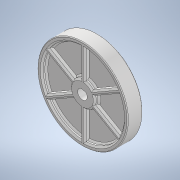
# Autodesk Inventor part: Test Gear
Saved by Autodesk Inventor 2020.2 (Build 242310000, 310)
## iProperties
Created: 2020-04-13
Part Number: Test Gear
Material: Generic
Document SubType Name: Modeling
Designer: Josiah
Density: 1 g/cm^3
Appearance: Default
Author: Josiah
Autodesk Inventor part; units mm, degrees
ref_plane "YZ Plane" through (0, 0, 0) normal (1, 0, 0) x (0, 1, 0)
ref_plane "XZ Plane" through (0, 0, 0) normal (0, 1, 0) x (-1, 0, 0)
ref_plane "XY Plane" through (0, 0, 0) normal (0, 0, 1) x (1, 0, 0)
sketch "Sketch1" plane through (0, 0, 0) normal (0, 0, 1) x (1, 0, 0)
  arc A0 (-1.6062, 0.3296) -> (1.6062, -0.4956) centre (-0.622, -2.5044) ccw
  line L0 (1.6062, -0.4956) -> (-1.6062, 0.3296)
  circle A1 centre (-0.622, -2.5044) radius 30
  arc A2 (-1.6138, 0.538) -> (1.7133, -0.3166) centre (-0.622, -2.5044) ccw
  line L1 (-1.6138, 0.538) -> (1.7133, -0.3166)
  point P0 (0, 0)
  dimension "d0" = 60
  dimension "d1" = 0.2
  constraints: 4 end point, 4 point on circle, 3 centre point, 1 coincident, 1 other
  measures "d0" diameter of A1
  measures "d1" radial gap between concentric circles of A0 A2
extrude "Extrusion1" add sketch "Sketch1" along normal blind 5 contours A1
sketch "Sketch2" plane through (-0.622, -2.5044, 5) normal (0, 0, 1) x (1, 0, 0)
  arc A0 (-0.9918, 3.0424) -> (2.3353, 2.1878) centre (0, 0) ccw projected
  line L0 (-0.9918, 3.0424) -> (2.3353, 2.1878) projected
  arc A1 (-0.8151, 8.1594) -> (4.6467, 6.7563) centre (0, 0) ccw
  circle A2 centre (0, 0) radius 30 projected
  circle A3 centre (0, 0) radius 27
  line L1 (1.5, -8.0616) -> (1.5, -26.9583)
  line L2 (-1.5, -8.0616) -> (-1.5, -26.9583)
  line L3 (0, 27) -> (0, -27) construction
  line L4 (6.2316, -5.3299) -> (22.5966, -14.7782)
  line L5 (7.7316, -2.7318) -> (24.0966, -12.1801)
  line L6 (7.7316, 2.7318) -> (24.0966, 12.1801)
  line L7 (6.2316, 5.3299) -> (22.5966, 14.7782)
  line L8 (1.5, 8.0616) -> (1.5, 26.9583)
  line L9 (-1.5, 8.0616) -> (-1.5, 26.9583)
  line L10 (-6.2316, 5.3299) -> (-22.5966, 14.7782)
  line L11 (-7.7316, 2.7318) -> (-24.0966, 12.1801)
  line L12 (-7.7316, -2.7318) -> (-24.0966, -12.1801)
  line L13 (-6.2316, -5.3299) -> (-22.5966, -14.7782)
  arc A4 (4.6467, 6.7563) -> (1.5, 8.0616) centre (0, 0) ccw
  point P0 (0.622, 2.5044)
  point P1 (24.0966, 12.1801)
  point P2 (24.0966, -12.1801)
  point P3 (22.5966, -14.7782)
  point P4 (-24.0966, -12.1801)
  point P5 (-24.0966, 12.1801)
  point P6 (-22.5966, 14.7782)
  dimension "d4" = 5
  dimension "d5" = 3
  dimension "d6" = 3
  dimension "d7" = 1.5
  dimension "d8" = 0
  dimension "d11" = 360
  constraints: 26 end point, 10 point on circle, 3 centre point, 2 parallel, 1 concentric, 1 vertical, 37 other
  measures "d4" radial gap between concentric circles of A0 A1
  measures "d5" radial gap between concentric circles of A2 A3
  measures "d6" distance between parallel lines of L2 L1
  measures "d7" distance between parallel lines of L1 L3
  measures "d8" distance from line of A0.centre L3
extrude "Extrusion2" cut sketch "Sketch2" against normal blind 3 contours A1 L10 A3 L9 | A1 L12 A3 L11 | A3 L7 A1 A4 L8 | A1 L2 A3 L13 | A3 L5 A1 L6 | A1 L4 A3 L1
chamfer "Chamfer1" distance 1 angle 45 24 edges at (-14.122, 20.8783, 5) (-2.122, 15.0056, 5) (-15.0361, 7.5496, 5) (0.878, 15.0056, 5) (12.878, 20.8783, 5) (13.7921, 7.5496, 5) (15.2921, 4.9516, 5) (26.378, -2.5044, 5) (15.2921, -9.9603, 5) (13.7921, -12.5584, 5) (12.878, -25.8871, 5) (0.878, -20.0144, 5) (-2.122, -20.0144, 5) (-4.722, -9.6058, 5) (-15.0361, -12.5584, 5) (-14.122, -25.8871, 5) (-27.622, -2.5044, 5) (-16.5361, -9.9603, 5) (-8.822, -2.5044, 5) (-16.5361, 4.9516, 5) (-4.722, 4.597, 5) (4.8637, 3.5904, 5) (7.578, -2.5044, 5) (3.478, -9.6058, 5)
chamfer "Chamfer2" distance 1 angle 45 12 edges at (-8.822, -2.5044, 2) (-4.722, -9.6058, 2) (3.478, -9.6058, 2) (7.578, -2.5044, 2) (4.8637, 3.5904, 2) (-4.722, 4.597, 2) (12.878, 20.8783, 2) (26.378, -2.5044, 2) (12.878, -25.8871, 2) (-14.122, -25.8871, 2) (-27.622, -2.5044, 2) (-14.122, 20.8783, 2)
fillet "Fillet1" radius 0.5 1 edges at (-30.622, -2.5044, 5)
mirror "Mirror2" about plane through (0, 0, 0) normal (0, 0, 1)
equation "\"d7\" = 0.5 * d6"
body "Solid1"
